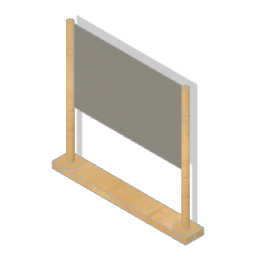
_Barrier, Pole and plate.243560d5-ae7e-49a1-a51b-d02f02e858bf (Autodesk Fusion 360 design; units mm, degrees)
Autodesk Fusion 360 part; units mm, degrees
sketch "Sketch1" plane through (0, 0, 0) normal (0, 0, 1) x (1, 0, 0)
  line L0 (0, 0) -> (-279.4, 0)
  line L1 (-279.4, 0) -> (-279.4, 38.1)
  line L2 (-279.4, 38.1) -> (0, 38.1)
  line L3 (0, 38.1) -> (0, 0)
  circle A0 centre (-260.35, 19.05) radius 19.05
  circle A1 centre (-19.05, 19.05) radius 19.05
  circle A2 centre (-260.35, 19.05) radius 6.35
  circle A3 centre (-19.05, 19.05) radius 6.35
  circle A4 centre (-260.35, 19.05) radius 15.875
  circle A5 centre (-19.05, 19.05) radius 15.875
  dimension "d1" = 279.4
  dimension "d2" = 38.1
  dimension "d3" = 12.7
  dimension "d4" = 12.7
  dimension "d5" = 31.75
  dimension "d6" = 31.75
  constraint horizontal L0
  constraint vertical L1
  constraint horizontal L2
  constraint vertical L3
  constraint coincident L0.start L3.end
  constraint tangent L0 A0
  constraint tangent L1 A0
  constraint tangent L2 A0
  constraint tangent L0 A1
  constraint tangent L3 A1
  constraint tangent L2 A1
  constraint concentric A0 A2
  constraint concentric A1 A3
  constraint concentric A2 A4
  constraint concentric A1 A5
  measures "d1" distance of L0.start L0.end
  measures "d2" distance of L0.start L2.end
  measures "d3" diameter of A2
  measures "d4" diameter of A3
  measures "d5" diameter of A4
  measures "d6" diameter of A5
extrude "Extrude1" add sketch "Sketch1" along normal blind 12.7 contours L0 L3 A1 | L0 L2 A0 A1 | L2 L3 A1 | L0 L1 A0 | L1 L2 A0 makes body 1 at (-173.5844, 19.5245, 0)
extrude "Extrude2" add sketch "Sketch1" along normal blind 9.525 separate body contours A1 | A0 | A2 | A3 | A4 | A5 makes body 2 at (-254.4933, 18.1036, 0) makes body 3 at (-0.0237, 18.1004, 3.175)
extrude "Extrude3" add sketch "Sketch1" against normal blind 254 contours A2 | A3 bodies 2 3
sketch "Sketch2" plane through (0, 0, -254) normal (0, 0, -1) x (1, 0, 0)
  circle A0 centre (-19.05, -19.05) radius 6.35
  line L0 (-253.7575, -18.6592) -> (-25.3948, -18.6592)
  line L1 (-25.3948, -18.6592) -> (-25.3948, -18.6846)
  line L2 (-25.3948, -18.6846) -> (-253.7575, -18.6846)
  line L3 (-253.7575, -18.6846) -> (-253.7575, -18.6592)
  dimension "d13" = 0.0254
  constraint horizontal L0
  constraint vertical L1
  constraint horizontal L2
  constraint vertical L3
  measures "d13" distance of L0.start L2.end
extrude "Extrude4" add sketch "Sketch2" against normal blind 152.4 separate body contours L0 L1 L2 L3 makes body 4
